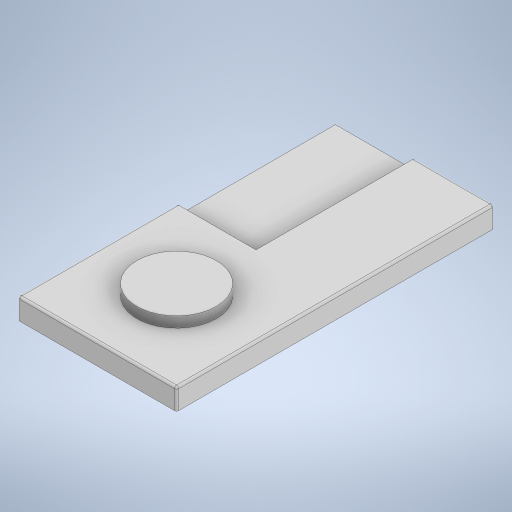
# Autodesk Inventor part: Body
Saved by Autodesk Inventor 2024.3 (Build 283343000, 343)
## iProperties
Created: 2024-08-06
Part Number: Body
Material: Generic
Document SubType Name: Modeling
Designer: lordk
Density: 1 g/cm^3
Appearance: Default
Author: lordk
Autodesk Inventor part; units mm, degrees
ref_plane "YZ Plane" through (0, 0, 0) normal (1, 0, 0) x (0, 1, 0)
ref_plane "XZ Plane" through (0, 0, 0) normal (0, 1, 0) x (-1, 0, 0)
ref_plane "XY Plane" through (0, 0, 0) normal (0, 0, 1) x (1, 0, 0)
sketch "Sketch3" plane through (0, 0, 0) normal (0, 1, 0) x (-1, 0, 0)
  line L0 (75, 150) -> (-75, 150)
  line L1 (-75, 150) -> (-75, -150)
  line L2 (-75, -150) -> (75, -150)
  line L3 (75, -150) -> (75, 150)
  line L4 (75, 150) -> (-75, -150) construction
  line L5 (-75, 150) -> (75, -150) construction
  point P0 (0, 0)
  dimension "d7" = 150
  dimension "d8" = 300
  constraints: 12 end point, 2 midpoint, 2 parallel, 1 horizontal, 1 perpendicular
  measures "d7" distance of L2.end L1.end
  measures "d8" distance of L1.end L0.end
extrude "Extrusion3" add sketch "Sketch3" along normal blind 20
sketch "Sketch4" plane through (0, 20, 0) normal (0, 1, 0) x (1, 0, 0)
  line L0 (75, 150) -> (-75, 150) projected
  line L1 (-75, 150) -> (0, 150)
  line L2 (0, 150) -> (0, 0)
  line L3 (0, 0) -> (-75, 0)
  line L4 (-75, 0) -> (-75, 150)
  dimension "d11" = 75
  dimension "d12" = 150
  constraints: 8 end point, 2 parallel, 1 horizontal, 1 perpendicular
  measures "d11" distance of L2.end L3.end
  measures "d12" distance of L1.end L2.end
extrude "Extrusion4" cut sketch "Sketch4" against normal blind 10
sketch "Sketch5" plane through (-75, 0, -150) normal (-1, 0, 0) x (0, 0, 1)
  line L0 (0, 0) -> (300, 0) projected
  line L1 (0, 0) -> (0, 10) projected
  line L2 (150, 20) -> (150, 10) projected
  point P0 (150, 0)
  point P1 (10, 5)
  point P2 (140, 5)
  dimension "d15" = 5
  dimension "d16" = 5
  dimension "d17" = 10
  dimension "d18" = 10
  measures "d15" distance from line of L0 point (10, 5)
  measures "d16" distance from line of L0 point (140, 5)
  measures "d17" distance from line of L1 point (10, 5)
  measures "d18" distance from line of L2 point (140, 5)
hole "Hole1" at (-75, 5, -10) at (-75, 5, -140) direction (1, 0, 0) diameter 3 depth 5 tip angle 118
fillet "Fillet1" radius 2 4 edges at (75, 20, 0) (0, 20, 150) (37.5, 20, -150) (-75, 20, 75)
fillet "Fillet2" radius 2 6 edges at (74.4142, 19.4142, 149.4142) (75, 9, 150) (-74.4142, 19.4142, 149.4142) (-75, 9, 150) (74.4142, 19.4142, -149.4142) (75, 9, -150)
sketch "Sketch6" plane through (0, 20, 0) normal (0, 1, 0) x (1, 0, 0)
  circle A0 centre (0, -75) radius 37.5
  line L0 (-73, -150) -> (73, -150) projected
  line L1 (-75, 0) -> (-75, -148) projected
  point P0 (0, 0)
  dimension "d28" = 75
  dimension "d29" = 75
  dimension "d30" = 75
  constraints: 1 centre point
  measures "d28" diameter of A0
  measures "d29" distance from line of L0 A0.centre
  measures "d30" distance from line of L1 A0.centre
extrude "Extrusion5" add sketch "Sketch6" along normal blind 10
body "Solid2"
